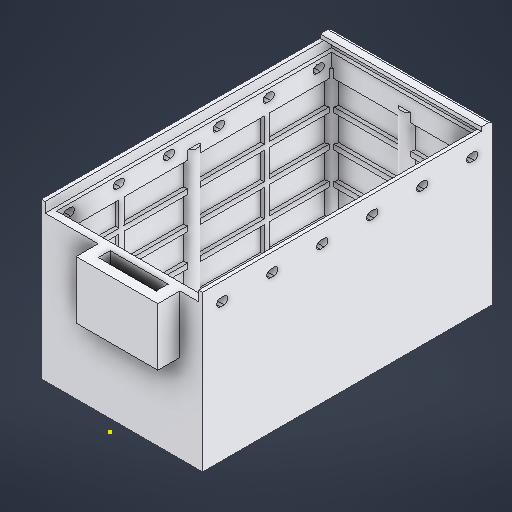
# Autodesk Inventor part: Caja con ranura
Saved by Autodesk Inventor 2026 (Build 300175000, 175)
## iProperties
Created: 2026-02-26
Part Number: Caja con ranura
Material: PET Plastic
Document SubType Name: Modeling
Designer: Usuario2
Density: 1.541 g/cm^3
Appearance: Weld - Aluminum
Mass: 81.677 g
Surface Area: 612.651 cm^2
Volume: 53.0026 cm^3
Author: Usuario2
Autodesk Inventor part; units mm, degrees
sketch "Sketch1" plane through (0, 0, 0) normal (0, 1, 0) x (-1, 0, 0)
  line L0 (31.75, 57.15) -> (-31.75, 57.15)
  line L1 (-31.75, 57.15) -> (-31.75, -57.15)
  line L2 (-31.75, -57.15) -> (31.75, -57.15)
  line L3 (31.75, -57.15) -> (31.75, 57.15)
  line L4 (31.75, 57.15) -> (-31.75, -57.15) construction
  line L5 (-31.75, 57.15) -> (31.75, -57.15) construction
  point P0 (0, 0)
  dimension "d0" = 63.5
  dimension "d1" = 114.3
  constraints: 12 end point, 2 midpoint, 2 parallel, 1 horizontal, 1 perpendicular
  measures "d0" distance of L2.end L1.end
  measures "d1" distance of L1.end L0.end
extrude "Extrusion1" add sketch "Sketch1" along normal blind 1.5
sketch "Sketch2" plane through (0, 1.5, 0) normal (0, 1, 0) x (1, 0, 0)
  line L0 (-31.75, 57.15) -> (31.75, 57.15)
  line L1 (31.75, 57.15) -> (31.75, -57.15)
  line L2 (31.75, -57.15) -> (-31.75, -57.15)
  line L3 (-31.75, -57.15) -> (-31.75, 57.15)
  line L4 (-31.75, 57.15) -> (31.75, -57.15) construction
  line L5 (31.75, 57.15) -> (-31.75, -57.15) construction
  line L6 (31.75, -57.15) -> (30.25, -57.15)
  line L7 (30.25, -57.15) -> (30.25, -55.65)
  line L8 (30.25, -55.65) -> (31.75, -55.65)
  line L9 (31.75, -55.65) -> (31.75, -57.15)
  line L10 (-31.75, 57.15) -> (-30.25, 57.15)
  line L11 (-30.25, 57.15) -> (-30.25, 55.65)
  line L12 (-30.25, 55.65) -> (-31.75, 55.65)
  line L13 (-31.75, 55.65) -> (-31.75, 57.15)
  line L14 (-30.25, 55.65) -> (30.25, 55.65)
  line L15 (30.25, 55.65) -> (30.25, -55.65)
  line L16 (30.25, -55.65) -> (-30.25, -55.65)
  line L17 (-30.25, -55.65) -> (-30.25, 55.65)
  point P0 (0, 0)
  dimension "d4" = 63.5
  dimension "d5" = 114.3
  dimension "d6" = 1.5
  dimension "d7" = 1.5
  dimension "d8" = 1.5
  dimension "d9" = 1.5
  constraints: 36 end point, 8 parallel, 4 horizontal, 4 perpendicular, 2 midpoint
  measures "d4" distance of L1.end L2.end
  measures "d5" distance of L0.end L1.end
  measures "d6" distance of L7.end L8.end
  measures "d7" distance of L6.end L7.end
  measures "d8" distance of L11.end L12.end
  measures "d9" distance of L10.end L11.end
extrude "Extrusion2" add sketch "Sketch2" along normal blind 50.8 contours L0 L11 L12 L3 | L0 L1 L8 L15 L14 L11 | L12 L17 L16 L7 L2 L3 | L1 L2 L7 L8
sketch "Sketch3" plane through (0, 1.5, 0) normal (0, 1, 0) x (1, 0, 0)
  line L0 (-30.25, -55.65) -> (-30.25, 55.65) projected
  line L1 (30.25, -55.65) -> (-30.25, -55.65)
  line L2 (-30.25, -55.65) -> (-30.25, 55.65)
  line L3 (-30.25, 55.65) -> (30.25, 55.65)
  line L4 (30.25, 55.65) -> (30.25, -55.65)
  line L5 (30.25, -55.65) -> (-30.25, 55.65) construction
  line L6 (-30.25, -55.65) -> (30.25, 55.65) construction
  line L7 (-30.25, -55.65) -> (-28.25, -55.65)
  line L8 (-28.25, -55.65) -> (-28.25, -53.65)
  line L9 (-28.25, -53.65) -> (-30.25, -53.65)
  line L10 (-30.25, -53.65) -> (-30.25, -55.65)
  circle A0 centre (-30.25, -55.65) radius 2.8284
  circle A1 centre (-30.25, 0.0014) radius 2.8284
  circle A2 centre (-30.25, 55.6528) radius 2.8284
  circle A3 centre (0.0014, -55.65) radius 2.8284
  circle A4 centre (0.0014, 0.0014) radius 2.8284
  circle A5 centre (0.0014, 55.6528) radius 2.8284
  circle A6 centre (30.2528, -55.65) radius 2.8284
  circle A7 centre (30.2528, 0.0014) radius 2.8284
  circle A8 centre (30.2528, 55.6528) radius 2.8284
  point P0 (0, 0)
  point P1 (-27.4216, -55.65)
  point P2 (-30.25, -52.8216)
  point P3 (-30.25, -55.65)
  point P4 (-28.25, 2.0014)
  point P5 (-28.25, 57.6528)
  point P6 (2.0014, -53.65)
  point P7 (2.0014, 2.0014)
  point P8 (2.0014, 57.6528)
  point P9 (32.2528, -53.65)
  point P10 (32.2528, 2.0014)
  point P11 (32.2528, 57.6528)
  point P12 (-30.25, 2.8298)
  point P13 (-30.25, -2.827)
  point P14 (-27.4216, 55.65)
  point P15 (-30.25, 52.8244)
  point P16 (-2.827, 55.65)
  point P17 (2.8298, 55.65)
  point P18 (27.4244, 55.65)
  point P19 (30.25, 52.8244)
  point P20 (30.25, -2.827)
  point P21 (30.25, 2.8298)
  point P22 (30.25, -52.8216)
  point P23 (27.4244, -55.65)
  point P24 (-2.827, -55.65)
  point P25 (2.8298, -55.65)
  point P26 (-30.25, 49.2176)
  point P27 (23.8176, -55.65)
  dimension "d12" = 2
  dimension "d13" = 2
  dimension "d18" = 55.6514
  dimension "d21" = 30.2514
  constraints: 20 end point, 9 horizontal, 4 parallel, 3 vertical, 2 midpoint, 2 perpendicular, 1 coincident, 43 other
  measures "d12" distance of L9.end L8.end
  measures "d13" distance of L8.end L7.end
  measures "d18" distance of point (-30.25, -55.65) point (-30.25, 0.001)
  measures "d21" distance of point (-30.25, -55.65) point (0.001, -55.65)
extrude "Extrusion3" add sketch "Sketch3" along normal blind 50.8 contours L0 L9 L8 L1 | L0 A0 L9 | L8 A0 L1 | L0 A1 | A3 L1 | L0 L3 A2 | A6 L4 L1 | L3 A5 | A7 L4 | L3 L4 A8 picked at (-29.3072, 0.0014) picked at (0.7071, -55.0248) picked at (-28.3882, 55.4404) picked at (30.0404, -53.7882) picked at (-0.1122, 54.715) picked at (29.315, -0.1122) picked at (30.0405, 53.7901)
ref_plane "Work Plane1" through (0, 12.7, 0) normal (0, -1, 0) x (1, 0, 0)
sketch "Sketch4" plane through (0, 12.7, 0) normal (0, -1, 0) x (1, 0, 0)
  line L0 (-31.75, 57.15) -> (31.75, 57.15)
  line L1 (31.75, 57.15) -> (31.75, -57.15)
  line L2 (31.75, -57.15) -> (-31.75, -57.15)
  line L3 (-31.75, -57.15) -> (-31.75, 57.15)
  line L4 (-31.75, 57.15) -> (31.75, -57.15) construction
  line L5 (31.75, 57.15) -> (-31.75, -57.15) construction
  line L6 (-31.75, -57.15) -> (-28.75, -57.15)
  line L7 (-28.75, -57.15) -> (-28.75, -54.15)
  line L8 (-28.75, -54.15) -> (-31.75, -54.15)
  line L9 (-31.75, -54.15) -> (-31.75, -57.15)
  line L10 (31.75, 57.15) -> (28.75, 57.15)
  line L11 (28.75, 57.15) -> (28.75, 54.15)
  line L12 (28.75, 54.15) -> (31.75, 54.15)
  line L13 (31.75, 54.15) -> (31.75, 57.15)
  line L14 (28.75, 54.15) -> (-28.75, 54.15)
  line L15 (-28.75, 54.15) -> (-28.75, -54.15)
  line L16 (-28.75, -54.15) -> (28.75, -54.15)
  line L17 (28.75, -54.15) -> (28.75, 54.15)
  point P0 (0, 0)
  dimension "d25" = 63.5
  dimension "d26" = 114.3
  dimension "d27" = 3
  dimension "d28" = 3
  dimension "d29" = 3
  dimension "d30" = 3
  constraints: 36 end point, 8 parallel, 4 horizontal, 4 perpendicular, 2 midpoint
  measures "d25" distance of L1.end L2.end
  measures "d26" distance of L0.end L1.end
  measures "d27" distance of L8.end L7.end
  measures "d28" distance of L7.end L6.end
  measures "d29" distance of L12.end L11.end
  measures "d30" distance of L11.end L10.end
extrude "Extrusion4" add sketch "Sketch4" along normal mid plane 2 contours L0 L11 L14 L15 L8 L3 | L0 L1 L12 L11 | L8 L7 L2 L3 | L12 L1 L2 L7 L16 L17
ref_plane "Work Plane2" through (0, 25.4, 0) normal (0, -1, 0) x (1, 0, 0)
sketch "Sketch5" plane through (0, 25.4, 0) normal (0, -1, 0) x (1, 0, 0)
  line L0 (31.75, -57.15) -> (-31.75, -57.15) projected
  line L1 (-31.75, 57.15) -> (31.75, 57.15)
  line L2 (31.75, 57.15) -> (31.75, -57.15)
  line L3 (31.75, -57.15) -> (-31.75, -57.15)
  line L4 (-31.75, -57.15) -> (-31.75, 57.15)
  line L5 (-31.75, 57.15) -> (31.75, -57.15) construction
  line L6 (31.75, 57.15) -> (-31.75, -57.15) construction
  line L7 (-28.75, -54.15) -> (28.75, -54.15)
  line L8 (28.75, -54.15) -> (28.75, 54.15)
  line L9 (28.75, 54.15) -> (-28.75, 54.15)
  line L10 (-28.75, 54.15) -> (-28.75, -54.15)
  line L11 (-28.75, -54.15) -> (28.75, 54.15) construction
  line L12 (28.75, -54.15) -> (-28.75, 54.15) construction
  point P0 (0, 0)
  dimension "d34" = 63.5
  dimension "d35" = 114.3
  dimension "d36" = 57.5
  dimension "d37" = 108.3
  constraints: 24 end point, 4 midpoint, 4 parallel, 2 horizontal, 2 perpendicular
  measures "d34" distance of L0.start L3.end
  measures "d35" distance of L1.end L0.start
  measures "d36" distance of L9.end L8.end
  measures "d37" distance of L8.end L7.end
extrude "Extrusion5" add sketch "Sketch5" along normal mid plane 2
ref_plane "Work Plane3" through (0, 38.1, 0) normal (0, -1, 0) x (1, 0, 0)
sketch "Sketch6" plane through (0, 38.1, 0) normal (0, -1, 0) x (1, 0, 0)
  line L0 (31.75, 57.15) -> (-31.75, 57.15)
  line L1 (-31.75, 57.15) -> (-31.75, -57.15)
  line L2 (-31.75, -57.15) -> (31.75, -57.15)
  line L3 (31.75, -57.15) -> (31.75, 57.15)
  line L4 (31.75, 57.15) -> (-31.75, -57.15) construction
  line L5 (-31.75, 57.15) -> (31.75, -57.15) construction
  line L6 (-28.75, 54.15) -> (28.75, 54.15)
  line L7 (28.75, 54.15) -> (28.75, -54.15)
  line L8 (28.75, -54.15) -> (-28.75, -54.15)
  line L9 (-28.75, -54.15) -> (-28.75, 54.15)
  line L10 (-28.75, 54.15) -> (28.75, -54.15) construction
  line L11 (28.75, 54.15) -> (-28.75, -54.15) construction
  point P0 (0, 0)
  dimension "d41" = 63.5
  dimension "d42" = 114.3
  dimension "d43" = 57.5
  dimension "d44" = 108.3
  constraints: 24 end point, 4 midpoint, 4 parallel, 2 horizontal, 2 perpendicular
  measures "d41" distance of L2.end L1.end
  measures "d42" distance of L1.end L0.end
  measures "d43" distance of L7.end L8.end
  measures "d44" distance of L6.end L7.end
extrude "Extrusion6" add sketch "Sketch6" along normal mid plane 2
ref_plane "Work Plane4" through (0, 50.8, 0) normal (0, -1, 0) x (1, 0, 0)
sketch "Sketch7" plane through (0, 50.8, 0) normal (0, -1, 0) x (1, 0, 0)
  line L0 (31.75, 57.15) -> (31.75, -57.15) projected
  line L1 (-31.75, 57.15) -> (31.75, 57.15)
  line L2 (31.75, 57.15) -> (31.75, -57.15)
  line L3 (31.75, -57.15) -> (-31.75, -57.15)
  line L4 (-31.75, -57.15) -> (-31.75, 57.15)
  line L5 (-31.75, 57.15) -> (31.75, -57.15) construction
  line L6 (31.75, 57.15) -> (-31.75, -57.15) construction
  line L7 (-28.75, 54.15) -> (28.75, 54.15)
  line L8 (28.75, 54.15) -> (28.75, -54.15)
  line L9 (28.75, -54.15) -> (-28.75, -54.15)
  line L10 (-28.75, -54.15) -> (-28.75, 54.15)
  line L11 (-28.75, 54.15) -> (28.75, -54.15) construction
  line L12 (28.75, 54.15) -> (-28.75, -54.15) construction
  point P0 (0, 0)
  point P1 (31.75, 57.15)
  dimension "d48" = 63.5
  dimension "d49" = 114.3
  dimension "d50" = 57.5
  dimension "d51" = 108.3
  constraints: 24 end point, 4 midpoint, 4 parallel, 2 horizontal, 2 perpendicular
  measures "d48" distance of L0.end L3.end
  measures "d49" distance of L1.end L0.end
  measures "d50" distance of L8.end L9.end
  measures "d51" distance of L7.end L8.end
extrude "Extrusion7" add sketch "Sketch7" along normal blind 2 and the other way blind 1.5
ref_plane "Work Plane5" through (-28.75, 0, -57.15) normal (-1, 0, 0) x (0, 0, 1)
ref_plane "Work Plane6" through (28.75, 0, 57.15) normal (1, 0, 0) x (0, 0, -1)
sketch "Sketch8" plane through (-31.75, 0, -57.15) normal (-1, 0, 0) x (0, 0, 1)
  line L0 (0, 0) -> (114.3, 0) projected
  line L1 (57.15, 0) -> (114.3, 0)
  line L2 (114.3, 0) -> (85.725, 0)
  line L3 (57.15, 0) -> (-0.1412, 0)
  line L4 (-0.1412, 0) -> (28.5044, 0)
  line L5 (28.5044, 0) -> (28.5044, 52.3)
  line L6 (54.7507, 52.3) -> (3.8951, 52.3) projected
  line L7 (85.725, 0) -> (85.725, 52.3)
  line L8 (86.725, 52.3) -> (84.725, 52.3)
  line L9 (84.725, 52.3) -> (84.725, 0)
  line L10 (84.725, 0) -> (86.725, 0)
  line L11 (86.725, 0) -> (86.725, 52.3)
  line L12 (86.725, 52.3) -> (84.725, 0) construction
  line L13 (84.725, 52.3) -> (86.725, 0) construction
  line L14 (29.5044, 52.3) -> (27.5044, 52.3)
  line L15 (27.5044, 52.3) -> (27.5044, 0)
  line L16 (27.5044, 0) -> (29.5044, 0)
  line L17 (29.5044, 0) -> (29.5044, 52.3)
  line L18 (29.5044, 52.3) -> (27.5044, 0) construction
  line L19 (27.5044, 52.3) -> (29.5044, 0) construction
  point P0 (85.725, 26.15)
  point P1 (28.5044, 26.15)
  point P2 (29.5044, 0)
  point P3 (29.5044, 52.3)
  point P4 (27.5044, 52.3)
  point P5 (27.5044, 0)
  dimension "d58" = 2
  dimension "d59" = 52.3
  dimension "d60" = 2
  dimension "d61" = 52.3
  constraints: 36 end point, 8 midpoint, 4 parallel, 3 perpendicular, 2 horizontal, 2 point on line, 1 collinear, 1 vertical
  measures "d58" distance of L10.end L9.end
  measures "d59" distance of L9.end L8.end
  measures "d60" distance of L16.end L15.end
  measures "d61" distance of L15.end L14.end
extrude "Extrusion8" add sketch "Sketch8" against normal blind 3
sketch "Sketch9" plane through (28.75, 0, 57.15) normal (1, 0, 0) x (0, 0, -1)
  line L0 (114.3, 0) -> (0, 0) projected
  line L1 (57.15, 0) -> (0, 0)
  line L2 (0, 0) -> (114.3, 0)
  line L3 (57.15, 0) -> (114.3, 0)
  line L4 (85.725, 0) -> (85.725, 52.3)
  line L5 (59.5493, 52.3) -> (110.4049, 52.3) projected
  line L6 (57.15, 0) -> (0, 0)
  line L7 (28.575, 0) -> (28.575, 52.3)
  line L8 (28.575, 0) -> (80.875, 0) construction
  line L9 (86.725, 52.3) -> (84.725, 52.3)
  line L10 (84.725, 52.3) -> (84.725, 0)
  line L11 (84.725, 0) -> (86.725, 0)
  line L12 (86.725, 0) -> (86.725, 52.3)
  line L13 (86.725, 52.3) -> (84.725, 0) construction
  line L14 (84.725, 52.3) -> (86.725, 0) construction
  line L15 (29.575, 52.3) -> (27.575, 52.3)
  line L16 (27.575, 52.3) -> (27.575, 0)
  line L17 (27.575, 0) -> (29.575, 0)
  line L18 (29.575, 0) -> (29.575, 52.3)
  line L19 (29.575, 52.3) -> (27.575, 0) construction
  line L20 (27.575, 52.3) -> (29.575, 0) construction
  point P0 (85.725, 26.15)
  point P1 (28.575, 26.15)
  point P2 (29.575, 0)
  point P3 (27.575, 0)
  dimension "d64" = 52.3
  dimension "d65" = 52.3
  dimension "d66" = 90
  dimension "d67" = 2
  dimension "d68" = 52.3
  dimension "d69" = 2
  dimension "d70" = 52.3
  constraints: 38 end point, 8 midpoint, 5 horizontal, 4 parallel, 3 perpendicular, 2 collinear, 1 point on line, 1 vertical
  measures "d64" distance of L4.start L4.end
  measures "d65" distance of L7.start L7.end
  measures "d66" angle of L8 L7
  measures "d67" distance of L11.end L10.end
  measures "d68" distance of L10.end L9.end
  measures "d69" distance of L17.end L16.end
  measures "d70" distance of L16.end L15.end
extrude "Extrusion9" add sketch "Sketch9" along normal blind 3
sketch "Sketch10" plane through (0, 52.3, 0) normal (0, 1, 0) x (1, 0, 0)
  line L0 (-31.75, -57.15) -> (31.75, -57.15) projected
  line L1 (31.75, 57.15) -> (-31.75, 57.15) projected
  line L2 (-31.75, -57.15) -> (31.75, -57.15)
  line L3 (31.75, -57.15) -> (31.75, 57.15)
  line L4 (31.75, 57.15) -> (-31.75, 57.15)
  line L5 (-31.75, 57.15) -> (-31.75, -57.15)
  arc A0 (-28.75, -53.2521) -> (-30.25, -52.8216) centre (-30.25, -55.65) ccw projected
  line L6 (-30.25, -55.65) -> (30.25, -55.65)
  line L7 (30.25, -55.65) -> (30.25, 55.65)
  line L8 (30.25, 55.65) -> (-30.25, 55.65)
  line L9 (-30.25, 55.65) -> (-30.25, -55.65)
  line L10 (-28.75, -54.15) -> (28.75, -54.15)
  line L11 (28.75, -54.15) -> (28.75, 54.15)
  line L12 (28.75, 54.15) -> (-28.75, 54.15)
  line L13 (-28.75, 54.15) -> (-28.75, -54.15)
  line L14 (-28.75, -54.15) -> (28.75, 54.15) construction
  line L15 (28.75, -54.15) -> (-28.75, 54.15) construction
  point P0 (0, 0)
  dimension "d73" = 60.5
  dimension "d74" = 111.3
  dimension "d75" = 108.3
  constraints: 28 end point, 6 parallel, 3 horizontal, 3 perpendicular, 2 midpoint
  measures "d73" distance of L8.end L7.end
  measures "d74" distance of L7.end L6.end
  measures "d75" distance of L11.end L10.end
extrude "Extrusion10" add sketch "Sketch10" along normal blind 5 contours L5 L1 L3 L0 | L9 L8 L7 L6
sketch "Sketch11" plane through (31.75, 0, 57.15) normal (1, 0, 0) x (0, 0, -1)
  line L0 (114.3, 0) -> (0, 0) projected
  line L1 (114.3, 57.3) -> (0, 57.3) projected
  line L2 (0, 0) -> (114.3, 0)
  line L3 (114.3, 0) -> (114.3, 57.3)
  line L4 (114.3, 57.3) -> (0, 57.3)
  line L5 (0, 57.3) -> (0, 0)
  line L6 (0, 57.3) -> (5, 57.3)
  line L7 (5, 57.3) -> (5, 52.3)
  line L8 (5, 52.3) -> (0, 52.3)
  line L9 (0, 52.3) -> (0, 57.3)
  line L10 (0, 57.3) -> (114.3, 57.3)
  line L11 (114.3, 57.3) -> (114.3, 52.3)
  line L12 (114.3, 52.3) -> (0, 52.3)
  line L13 (0, 52.3) -> (0, 57.3)
  line L14 (5, 52.3) -> (9, 52.3)
  line L15 (9, 52.3) -> (9, 54.3)
  line L16 (9, 54.3) -> (5, 54.3)
  line L17 (5, 54.3) -> (5, 52.3)
  circle A0 centre (7, 54.3) radius 1.5
  line L18 (7, 54.3) -> (8.5, 54.3)
  circle A1 centre (8.5, 54.3) radius 1.5
  line L19 (7, 54.3) -> (7, 55.8)
  line L20 (7, 55.8) -> (8.5, 55.8)
  line L21 (7, 54.3) -> (7, 52.8)
  line L22 (7, 52.8) -> (8.5, 52.8)
  line L23 (26.7, 54.3) -> (28.2, 54.3)
  line L24 (26.7, 52.8) -> (28.2, 52.8)
  circle A2 centre (26.7, 54.3) radius 1.5
  circle A3 centre (28.2, 54.3) radius 1.5
  line L25 (24.7, 54.3) -> (24.7, 52.3)
  line L26 (24.7, 57.3) -> (24.7, 52.3)
  line L27 (28.7, 52.3) -> (28.7, 54.3)
  line L28 (24.7, 52.3) -> (28.7, 52.3)
  line L29 (24.7, 52.3) -> (19.7, 52.3)
  line L30 (28.7, 54.3) -> (24.7, 54.3)
  line L31 (26.7, 55.8) -> (28.2, 55.8)
  line L32 (26.7, 54.3) -> (26.7, 55.8)
  line L33 (26.7, 54.3) -> (26.7, 52.8)
  line L34 (19.7, 57.3) -> (24.7, 57.3)
  line L35 (19.7, 52.3) -> (19.7, 57.3)
  line L36 (19.7, 52.3) -> (19.7, 57.3)
  line L37 (46.4, 54.3) -> (47.9, 54.3)
  line L38 (46.4, 52.8) -> (47.9, 52.8)
  circle A4 centre (46.4, 54.3) radius 1.5
  circle A5 centre (47.9, 54.3) radius 1.5
  line L39 (44.4, 54.3) -> (44.4, 52.3)
  line L40 (44.4, 57.3) -> (44.4, 52.3)
  line L41 (48.4, 52.3) -> (48.4, 54.3)
  line L42 (44.4, 52.3) -> (48.4, 52.3)
  line L43 (44.4, 52.3) -> (39.4, 52.3)
  line L44 (48.4, 54.3) -> (44.4, 54.3)
  line L45 (46.4, 55.8) -> (47.9, 55.8)
  line L46 (46.4, 54.3) -> (46.4, 55.8)
  line L47 (46.4, 54.3) -> (46.4, 52.8)
  line L48 (39.4, 57.3) -> (44.4, 57.3)
  line L49 (39.4, 52.3) -> (39.4, 57.3)
  line L50 (39.4, 52.3) -> (39.4, 57.3)
  line L51 (66.1, 54.3) -> (67.6, 54.3)
  line L52 (66.1, 52.8) -> (67.6, 52.8)
  circle A6 centre (66.1, 54.3) radius 1.5
  circle A7 centre (67.6, 54.3) radius 1.5
  line L53 (64.1, 54.3) -> (64.1, 52.3)
  line L54 (64.1, 57.3) -> (64.1, 52.3)
  line L55 (68.1, 52.3) -> (68.1, 54.3)
  line L56 (64.1, 52.3) -> (68.1, 52.3)
  line L57 (64.1, 52.3) -> (59.1, 52.3)
  line L58 (68.1, 54.3) -> (64.1, 54.3)
  line L59 (66.1, 55.8) -> (67.6, 55.8)
  line L60 (66.1, 54.3) -> (66.1, 55.8)
  line L61 (66.1, 54.3) -> (66.1, 52.8)
  line L62 (59.1, 57.3) -> (64.1, 57.3)
  line L63 (59.1, 52.3) -> (59.1, 57.3)
  line L64 (59.1, 52.3) -> (59.1, 57.3)
  line L65 (85.8, 54.3) -> (87.3, 54.3)
  line L66 (85.8, 52.8) -> (87.3, 52.8)
  circle A8 centre (85.8, 54.3) radius 1.5
  circle A9 centre (87.3, 54.3) radius 1.5
  line L67 (83.8, 54.3) -> (83.8, 52.3)
  line L68 (83.8, 57.3) -> (83.8, 52.3)
  line L69 (87.8, 52.3) -> (87.8, 54.3)
  line L70 (83.8, 52.3) -> (87.8, 52.3)
  line L71 (83.8, 52.3) -> (78.8, 52.3)
  line L72 (87.8, 54.3) -> (83.8, 54.3)
  line L73 (85.8, 55.8) -> (87.3, 55.8)
  line L74 (85.8, 54.3) -> (85.8, 55.8)
  line L75 (85.8, 54.3) -> (85.8, 52.8)
  line L76 (78.8, 57.3) -> (83.8, 57.3)
  line L77 (78.8, 52.3) -> (78.8, 57.3)
  line L78 (78.8, 52.3) -> (78.8, 57.3)
  line L79 (105.5, 54.3) -> (107, 54.3)
  line L80 (105.5, 52.8) -> (107, 52.8)
  circle A10 centre (105.5, 54.3) radius 1.5
  circle A11 centre (107, 54.3) radius 1.5
  line L81 (103.5, 54.3) -> (103.5, 52.3)
  line L82 (103.5, 57.3) -> (103.5, 52.3)
  line L83 (107.5, 52.3) -> (107.5, 54.3)
  line L84 (103.5, 52.3) -> (107.5, 52.3)
  line L85 (103.5, 52.3) -> (98.5, 52.3)
  line L86 (107.5, 54.3) -> (103.5, 54.3)
  line L87 (105.5, 55.8) -> (107, 55.8)
  line L88 (105.5, 54.3) -> (105.5, 55.8)
  line L89 (105.5, 54.3) -> (105.5, 52.8)
  line L90 (98.5, 57.3) -> (103.5, 57.3)
  line L91 (98.5, 52.3) -> (98.5, 57.3)
  line L92 (98.5, 52.3) -> (98.5, 57.3)
  point P0 (57.15, 0)
  point P1 (19.7, 57.3)
  point P2 (39.4, 57.3)
  point P3 (59.1, 57.3)
  point P4 (78.8, 57.3)
  point P5 (98.5, 57.3)
  dimension "d78" = 114.3
  dimension "d79" = 57.3
  dimension "d80" = 5
  dimension "d81" = 5
  dimension "d82" = 5
  dimension "d83" = 4
  dimension "d84" = 2
  dimension "d85" = 3
  dimension "d86" = 1.5
  dimension "d87" = 3
  dimension "d90" = 19.7
  constraints: 182 end point, 24 point on circle, 13 point on line, 12 centre point, 8 parallel, 6 coincident, 5 horizontal, 5 perpendicular, 2 tangent, 1 midpoint, 160 other
  measures "d78" distance of L4.end L1.start
  measures "d79" distance of L1.start L2.end
  measures "d80" distance of L7.end L8.end
  measures "d81" distance of L6.end L7.end
  measures "d82" distance of L10.end L11.end
  measures "d83" distance of L16.end L15.end
  measures "d84" distance of L15.end L14.end
  measures "d85" diameter of A0
  measures "d86" distance of L18.start L18.end
  measures "d87" diameter of A1
  measures "d90" distance of L16.end L25.start
extrude "Extrusion11" cut sketch "Sketch11" against normal through all contours L83 L86 A10 A11 | A11 A10 L86 L83 | L80 A10 A11 | A0 L19 L16 | L16 L21 A0 | A1 A0 L16 L15 | L15 L16 A0 A1 | L86 L89 A10 | A10 L88 L86 | L89 A11 A10 | A11 L79 A10 | A11 A10 L87 | L79 A11 A10 | A1 A0 L16 | L19 A0 A1 | L16 A0 A1 | A1 A0 L21 | L20 A1 A0 | A0 A1 L22 | A10 A11 L88 | L69 L72 A8 A9 | A9 A8 L72 L69 | L72 L75 A8 | A8 L74 L72 | L66 A8 A9 | L30 L33 A2 | A2 L32 L30 | L27 L30 A2 A3 | A3 A2 L30 L27 | L73 A9 A8 | A8 A9 L74 | L75 A9 A8 | A9 A8 L65 | L65 A8 A9 | L31 A3 A2 | A2 A3 L32 | A2 A3 L24 | L33 A3 A2 | A3 A2 L23 | L23 A2 A3 | L58 L61 A6 | A6 L60 L58 | L55 L58 A6 A7 | A7 A6 L58 L55 | L44 L47 A4 | A4 L46 L44 | L59 A7 A6 | A6 A7 L60 | A6 A7 L52 | L61 A7 A6 | A7 A6 L51 | L51 A6 A7 | L45 A5 A4 | A4 A5 L46 | A4 A5 L38 | L47 A5 A4 | A5 A4 L37 | L37 A4 A5 | L41 L44 A4 A5 | A5 A4 L44 L41
sketch "Sketch12" plane through (0, 57.3, 0) normal (0, 1, 0) x (1, 0, 0)
  line L0 (30.25, -54.15) -> (-30.25, -54.15)
  line L1 (-30.25, -54.15) -> (-30.25, 54.15)
  line L2 (-30.25, 54.15) -> (30.25, 54.15)
  line L3 (30.25, 54.15) -> (30.25, -54.15)
  line L4 (30.25, -54.15) -> (-30.25, 54.15) construction
  line L5 (-30.25, -54.15) -> (30.25, 54.15) construction
  line L6 (-31.75, -57.15) -> (31.75, -57.15) projected
  line L7 (30.25, -54.15) -> (30.25, -57.15)
  line L8 (-30.25, 54.15) -> (-30.25, 57.15)
  line L9 (31.75, 57.15) -> (-31.75, 57.15) projected
  line L10 (30.25, 54.15) -> (30.25, 57.15)
  line L11 (-30.25, -54.15) -> (-31.75, -54.15)
  line L12 (-31.75, -54.15) -> (-31.75, -57.15)
  line L13 (-31.75, -57.15) -> (-30.25, -57.15)
  line L14 (-30.25, -57.15) -> (-30.25, -54.15)
  line L15 (-31.75, 57.15) -> (31.9259, 57.15)
  line L16 (31.9259, 57.15) -> (31.9259, -57.15)
  line L17 (31.9259, -57.15) -> (-31.75, -57.15)
  line L18 (-31.75, -57.15) -> (-31.75, 57.15)
  line L19 (-30.25, 54.15) -> (-31.75, 54.15)
  line L20 (-31.75, 54.15) -> (-31.75, 57.15)
  line L21 (-31.75, 57.15) -> (-30.25, 57.15)
  line L22 (-30.25, 57.15) -> (-30.25, 54.15)
  line L23 (31.75, -57.15) -> (31.75, 57.15) projected
  line L24 (30.25, -54.15) -> (31.75, -54.15)
  line L25 (31.75, -54.15) -> (31.75, -57.15)
  line L26 (31.75, -57.15) -> (30.25, -57.15)
  line L27 (30.25, -57.15) -> (30.25, -54.15)
  line L28 (30.25, 54.15) -> (31.75, 54.15)
  line L29 (31.75, 54.15) -> (31.75, 57.15)
  line L30 (31.75, 57.15) -> (30.25, 57.15)
  line L31 (30.25, 57.15) -> (30.25, 54.15)
  line L32 (-30.25, 57.15) -> (30.25, 57.15)
  line L33 (30.25, 57.15) -> (30.25, 55.65)
  line L34 (30.25, 55.65) -> (-30.25, 55.65)
  line L35 (-30.25, 55.65) -> (-30.25, 57.15)
  point P0 (0, 0)
  dimension "d97" = 60.5
  dimension "d100" = 1.5
  constraints: 66 end point, 14 parallel, 8 perpendicular, 7 horizontal, 5 point on line, 3 midpoint, 1 vertical
  measures "d97" distance of L1.end L2.end
  measures "d100" distance of L32.end L33.end
extrude "Extrusion12" add sketch "Sketch12" along normal blind 4 contours L24 L23 L6 L7 | L3 L28 L23 L24 | L11 L18 L19 L1 | L14 L6 L12 L11 | L10 L9 L23 L28 | L19 L18 L9 L8 | L34 L8 L9 L10
ref_plane "Work Plane7" through (-31.75, 0, 57.15) normal (0, 0, 1) x (1, 0, 0)
sketch "Sketch13" plane through (-31.75, 0, 57.15) normal (0, 0, 1) x (1, 0, 0)
  line L0 (63.5, 0) -> (63.5, 61.3) projected
  line L1 (0, 0) -> (63.5, 0)
  line L2 (63.5, 0) -> (63.5, 61.3)
  line L3 (63.5, 61.3) -> (0, 61.3)
  line L4 (0, 61.3) -> (0, 0)
  line L5 (0, 61.3) -> (31.75, 61.3)
  line L6 (63.5, 61.3) -> (0, 61.3) projected
  line L7 (31.75, 0) -> (31.75, 61.3)
  line L8 (31.75, 61.3) -> (31.75, 34.6)
  line L9 (31.75, 34.6) -> (38.5, 34.6)
  line L10 (34.5798, 37.1) -> (34.5798, 26.4) projected
  line L11 (31.75, 34.6) -> (38.5, 34.6) construction
  line L12 (38.5, 34.6) -> (54.6, 34.6)
  line L13 (54.6, 34.6) -> (54.6, 61.3)
  line L14 (54.6, 61.3) -> (38.5, 61.3)
  line L15 (38.5, 61.3) -> (38.5, 34.6)
  line L16 (38.5, 34.6) -> (22.4, 34.6)
  line L17 (22.4, 34.6) -> (22.4, 61.3)
  line L18 (22.4, 61.3) -> (38.5, 61.3)
  line L19 (38.5, 61.3) -> (38.5, 34.6)
  line L20 (54.6, 61.3) -> (49.9, 61.3)
  line L21 (49.9, 61.3) -> (49.9, 34.6)
  line L22 (49.9, 34.6) -> (54.6, 34.6)
  line L23 (54.6, 34.6) -> (54.6, 61.3)
  line L24 (22.4, 61.3) -> (27.1, 61.3)
  line L25 (27.1, 61.3) -> (27.1, 34.6)
  line L26 (27.1, 34.6) -> (22.4, 34.6)
  line L27 (22.4, 34.6) -> (22.4, 61.3)
  line L28 (1.5, 57.3) -> (62, 57.3) projected
  line L29 (22.4, 61.3) -> (54.6, 61.3)
  line L30 (54.6, 61.3) -> (54.6, 57.3)
  line L31 (54.6, 57.3) -> (22.4, 57.3)
  line L32 (22.4, 57.3) -> (22.4, 61.3)
  point P0 (27.1, 57.3)
  point P1 (49.9, 57.3)
  dimension "d119" = 26.7
  dimension "d120" = 6.75
  dimension "d121" = 0
  dimension "d122" = 16.1
  dimension "d123" = 16.1
  dimension "d124" = 4.7
  dimension "d125" = 4.7
  constraints: 58 end point, 13 parallel, 7 horizontal, 7 perpendicular, 7 point on line, 1 collinear, 1 midpoint
  measures "d119" distance of L5.end L8.end
  measures "d120" distance of L8.end L9.end
  measures "d121" distance between parallel lines of L9 L11
  measures "d122" distance of L14.end L13.end
  measures "d123" distance of L17.end L18.end
  measures "d124" distance of L22.end L21.end
  measures "d125" distance of L25.end L26.end
ref_plane "Work Plane8" through (0, 61.3, 0) normal (0, 1, 0) x (1, 0, 0)
sketch "Sketch15" plane through (0, 61.3, 0) normal (0, 1, 0) x (1, 0, 0)
  line L0 (31.75, 57.15) -> (-31.75, 57.15) projected
  line L1 (-31.75, -57.15) -> (31.75, -57.15)
  line L2 (31.75, -57.15) -> (31.75, 57.15)
  line L3 (31.75, 57.15) -> (-31.75, 57.15)
  line L4 (-31.75, 57.15) -> (-31.75, -57.15)
  line L5 (-31.75, -57.15) -> (31.75, 57.15) construction
  line L6 (31.75, -57.15) -> (-31.75, 57.15) construction
  line L7 (-28.75, -54.15) -> (28.75, -54.15)
  line L8 (28.75, -54.15) -> (28.75, 54.15)
  line L9 (28.75, 54.15) -> (-28.75, 54.15)
  line L10 (-28.75, 54.15) -> (-28.75, -54.15)
  line L11 (-28.75, -54.15) -> (28.75, 54.15) construction
  line L12 (28.75, -54.15) -> (-28.75, 54.15) construction
  line L13 (28.75, 54.15) -> (31.75, 54.15)
  line L14 (-28.75, 54.15) -> (-31.75, 54.15)
  line L15 (31.75, -57.15) -> (31.75, 57.15) projected
  line L16 (-31.75, 57.15) -> (31.75, 57.15)
  line L17 (31.75, 57.15) -> (31.75, 55.65)
  line L18 (31.75, 55.65) -> (-31.75, 55.65)
  line L19 (-31.75, 55.65) -> (-31.75, 57.15)
  point P0 (0, 0)
  point P1 (-31.75, 55.65)
  dimension "d103" = 1.5
  constraints: 36 end point, 6 parallel, 5 point on line, 4 midpoint, 3 horizontal, 3 perpendicular
  measures "d103" distance of L16.end L17.end
revolve "Revolution1" add sketch "Sketch15" angle 90 about axis through (31.75, 61.3, -55.65) along (1, 0, 0) contours L2 L18 L4 L0
sketch "Sketch16" plane through (-30.25, 57.3, -55.65) normal (0, 0, 1) x (1, 0, 0)
  line L0 (0, 0) -> (0, 4) projected
  line L1 (0, 0) -> (0, 5.5)
  line L2 (62, 5.5) -> (-1.5, 5.5) projected
  line L3 (-1.5, 5.5) -> (-1.5, 4) projected
  line L4 (0, 5.5) -> (-1.5, 5.5)
  line L5 (-1.5, 5.5) -> (-1.5, 4)
  line L6 (-1.5, 4) -> (0, 4)
  line L7 (0, 4) -> (0, 5.5)
  line L8 (62, 4) -> (60.5, 4) projected
  line L9 (0, 5.5) -> (62, 5.5)
  line L10 (62, 5.5) -> (62, 4)
  line L11 (62, 4) -> (0, 4)
  line L12 (0, 4) -> (0, 5.5)
  point P0 (30.25, -57.3)
  dimension "d105" = 5.5
  constraints: 18 end point, 4 parallel, 2 horizontal, 2 perpendicular, 1 point on line
  measures "d105" distance of L0.start L1.end
extrude "Extrusion13" add sketch "Sketch16" along normal blind 3
extrude "Extrusion14" add sketch "Sketch13" along normal blind 4.8 contours L13 L12 L21 L28 | L16 L17 L28 L25
sketch "Sketch17" plane through (-31.75, 0, 61.95) normal (0, 0, 1) x (1, 0, 0)
  point P0 (31.75, 0)
ref_plane "Work Plane9" through (-31.75, 0, 61.85) normal (0, 0, 1) x (1, 0, 0)
sketch "Sketch18" plane through (-31.75, 0, 61.85) normal (0, 0, 1) x (1, 0, 0)
  line L0 (63.5, 61.3) -> (63.5, 62.8) projected
  line L1 (0, 0) -> (63.5, 0)
  line L2 (63.5, 0) -> (63.5, 62.8)
  line L3 (63.5, 62.8) -> (0, 62.8)
  line L4 (0, 62.8) -> (0, 0)
  line L5 (22.4, 57.3) -> (22.4, 34.6) projected
  line L6 (54.6, 57.3) -> (54.6, 34.6) projected
  line L7 (22.4, 34.6) -> (54.6, 34.6)
  line L8 (54.6, 34.6) -> (54.6, 57.3)
  line L9 (54.6, 57.3) -> (22.4, 57.3)
  line L10 (22.4, 57.3) -> (22.4, 34.6)
  point P0 (31.75, 0)
  constraints: 16 end point, 4 parallel, 2 horizontal, 2 perpendicular
extrude "Extrusion15" add sketch "Sketch18" along normal blind 4 contours L9 L6 L7 L5
body "Solid1"
